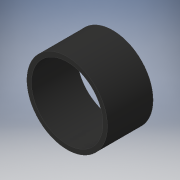
# Autodesk Inventor part: wheel ring
Saved by Autodesk Inventor 2018 (Build 220112000, 112)
## iProperties
Created: 2017-11-23
Part Number: wheel ring
Material: Rubber
Document SubType Name: Modeling
Designer: prakh
Density: 0.93 g/cm^3
Appearance: Rubber - Black
Author: prakh
Autodesk Inventor part; units mm, degrees
ref_plane "YZ Plane" through (0, 0, 0) normal (1, 0, 0) x (0, 1, 0)
ref_plane "XZ Plane" through (0, 0, 0) normal (0, 1, 0) x (-1, 0, 0)
ref_plane "XY Plane" through (0, 0, 0) normal (0, 0, 1) x (1, 0, 0)
sketch "Sketch1" plane through (0, 0, 0) normal (0, 0, 1) x (1, 0, 0)
  circle A0 centre (0, 0) radius 57.15
  circle A1 centre (0, 0) radius 50.8
  dimension "d1" = 6.35
  dimension "d4" = 101.6
  constraints: 2 centre point, 2 coincident
  measures "d1" radial gap between concentric circles of A0 A1
  measures "d4" diameter of A1
extrude "Extrusion1" add sketch "Sketch1" along normal blind 64.77
body "Solid1"
